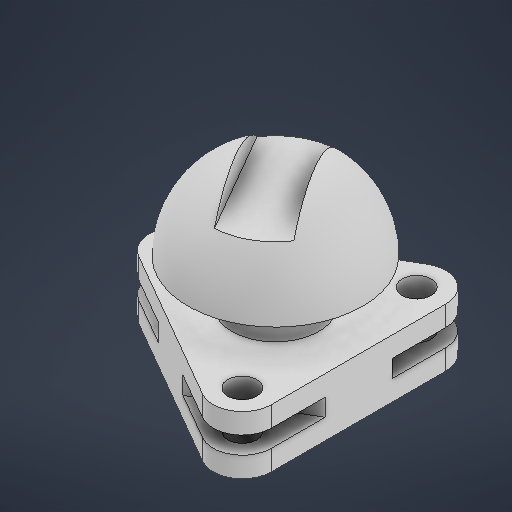
# Autodesk Inventor part: b4
Saved by Autodesk Inventor 2025.4 (Build 294407000, 407)
## iProperties
Created: 2026-05-15
Part Number: b4
Material: Generic
Document SubType Name: Modeling
Designer: VuQuan
Density: 1 g/cm^3
Appearance: Default
Author: VuQuan
Autodesk Inventor part; units mm, degrees
ref_plane "YZ Plane" through (0, 0, 0) normal (1, 0, 0) x (0, 1, 0)
ref_plane "XZ Plane" through (0, 0, 0) normal (0, 1, 0) x (-1, 0, 0)
sketch "Sketch1" plane through (0, 0, 0) normal (0, 1, 0) x (-1, 0, 0)
  line L0 (79.282, -17.3205) -> (-24.641, -77.3205)
  line L1 (-54.641, -60) -> (-54.641, 60)
  line L2 (-24.641, 77.3205) -> (79.282, 17.3205)
  arc A0 (79.282, -17.3205) -> (79.282, 17.3205) centre (69.282, 0) ccw
  arc A1 (-54.641, -60) -> (-24.641, -77.3205) centre (-34.641, -60) ccw
  arc A2 (-24.641, 77.3205) -> (-54.641, 60) centre (-34.641, 60) ccw
  line L3 (47.282, -35.7957) -> (47.282, 35.7957)
  line L4 (7.359, 58.8453) -> (-54.641, 23.0496)
  line L5 (-54.641, -23.0496) -> (7.359, -58.8453)
  circle A3 centre (69.282, 0) radius 10
  circle A4 centre (-34.641, -60) radius 10
  circle A5 centre (-34.641, 60) radius 10
  point P0 (0, 0)
  point P1 (109.282, 0)
  point P2 (-54.641, -94.641)
  point P3 (-54.641, 94.641)
  point P4 (0, 0)
  dimension "d18" = 20
  dimension "d19" = 120
  dimension "d22" = 22
  dimension "d25" = 360
  dimension "d27" = 20
  constraints: 12 end point, 8 point on line, 6 centre point, 6 point on circle, 6 tangent, 4 coincident, 4 equal radius, 1 parallel, 1 vertical, 17 other
  measures "d18" radius of A0
  measures "d19" distance of A1.centre A2.centre
  measures "d22" distance from line of L3 A0.centre
  measures "d27" diameter of A3
extrude "Extrusion1" add sketch "Sketch1" along normal blind 40 contours L0 L5 L1 L4 L2 L3
extrude "Extrusion2" add sketch "Sketch1" along normal blind 14 contours L4 L1 A2 L2
extrude "Extrusion3" add sketch "Sketch1" against normal blind 14 from surface at 40 contours L4 L1 A2 L2
pattern_circular "Circular Pattern1" count 3 over 360 about axis through (0, -10, 0) along (0, 1, 0) of "Extrusion3", "Extrusion2"
ref_plane "Work Plane1" through (0, 70, 0) normal (0, 1, 0) x (1, 0, 0)
sketch "Sketch2" plane through (0, 70, 0) normal (0, 1, 0) x (1, 0, 0)
  line L0 (54.641, 60) -> (54.641, -60) projected
  line L1 (-79.282, 17.3205) -> (24.641, 77.3205) projected
  line L2 (24.641, -77.3205) -> (-79.282, -17.3205) projected
  circle A0 centre (-2.6063, 0) radius 57.2473
  circle A1 centre (-2.6063, 0) radius 30
  point P0 (0, 0)
  point P1 (-7.359, 58.8453)
  point P2 (-47.282, 35.7957)
  point P3 (-47.282, -35.7957)
  point P4 (-7.359, -58.8453)
  dimension "d38" = 60
  constraints: 2 centre point, 2 point on circle, 1 coincident, 1 tangent
  measures "d38" diameter of A1
extrude "Extrusion4" add sketch "Sketch2" against normal up to surface (30 mm away) contours A1
sketch "Sketch3" plane through (0, 0, 0) normal (0, 0, 1) x (1, 0, 0)
  line L0 (27.3937, 70) -> (-32.6063, 70) projected
  line L1 (57.3937, 70) -> (-2.6063, 70)
  line L2 (-2.6063, 70) -> (-2.6063, 130)
  arc A0 (57.3937, 70) -> (-2.6063, 130) centre (-2.6063, 70) ccw
  line L3 (-32.6063, 40) -> (27.3937, 40) projected
  point P0 (0, 0)
  point P1 (-2.6063, 70)
  dimension "d41" = 60
  constraints: 4 end point, 2 midpoint, 2 point on circle, 2 point on line, 1 centre point, 1 vertical
  measures "d41" radius of A0
revolve "Revolution1" add sketch "Sketch3" angle 360 about axis through (-2.6063, 70, 0) along (0, 1, 0)
sketch "Sketch4" plane through (-79.282, 0, -17.3205) normal (-0.5, 0, -0.8660254) x (-0.8660254, 0, 0.5)
  arc A0 (2.2571, 70) -> (-117.7429, 70) centre (-57.7429, 70) ccw projected
  line L0 (-77.7429, 126.5685) -> (-77.7429, 110)
  line L1 (-77.7429, 110) -> (-37.7429, 110)
  line L2 (-37.7429, 110) -> (-37.7429, 126.5685)
  line L3 (2.2571, 70) -> (-117.7429, 70) projected
  point P0 (-60, 0)
  dimension "d43" = 40
  dimension "d44" = 40
  constraints: 6 end point, 2 point on circle, 1 horizontal, 1 parallel, 1 perpendicular, 1 vertical
  measures "d43" distance between parallel lines of L2 L0
  measures "d44" distance between parallel lines of L3 L1
extrude "Extrusion5" cut sketch "Sketch4" against normal up to surface contours L2 L1 L0 A0
body "Solid1"
